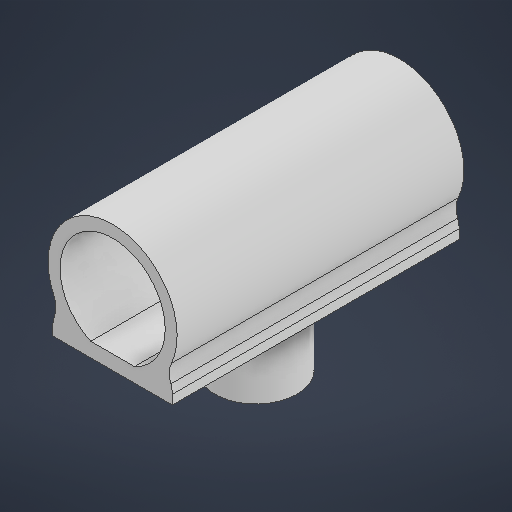
# Autodesk Inventor part: wire_loop
Saved by Autodesk Inventor 2027 (Build 310192060, 192F)
## iProperties
Created: 2026-07-23
Part Number: wire_loop
Material: Ogólny
Document SubType Name: Modeling
Designer: User
Density: 1 g/cm^3
Appearance: Domyślna
Author: User
Autodesk Inventor part; units mm, degrees
ref_plane "YZ Plane" through (0, 0, 0) normal (1, 0, 0) x (0, 1, 0)
ref_plane "XZ Plane" through (0, 0, 0) normal (0, 1, 0) x (-1, 0, 0)
ref_plane "XY Plane" through (0, 0, 0) normal (0, 0, 1) x (1, 0, 0)
sketch "Szkic1" plane through (0, 0, 0) normal (0, 1, 0) x (-1, 0, 0)
  circle A0 centre (0, 0) radius 1.72
  line L0 (-2.5, 6) -> (2.5, 6)
  line L1 (2.5, 6) -> (2.5, -6)
  line L2 (2.5, -6) -> (-2.5, -6)
  line L3 (-2.5, -6) -> (-2.5, 6)
  line L4 (-2.5, 6) -> (2.5, -6) construction
  line L5 (2.5, 6) -> (-2.5, -6) construction
  dimension "d0" = 3.44
  dimension "d1" = 5
  dimension "d2" = 12
  constraints: 12 end point, 2 midpoint, 2 parallel, 1 centre point, 1 coincident, 1 horizontal, 1 perpendicular
  measures "d0" diameter of A0
  measures "d1" distance of L1.end L2.end
  measures "d2" distance of L0.end L1.end
extrude "Wyciągnięcie proste1" add sketch "Szkic1" against normal blind 3 contours A0
extrude "Wyciągnięcie proste2" add sketch "Szkic1" along normal blind 0.6 contours A0 | L0 L1 L2 L3
sketch "Szkic2" plane through (-2.5, 0, 6) normal (0, 0, 1) x (1, 0, 0)
  line L0 (5, 0.6) -> (0, 0.6) projected
  line L1 (2.5, 0.6) -> (2.5, 2.6)
  line L2 (2.5, 0.6) -> (4.5, 0.6) construction
  circle A0 centre (2.5, 2.6) radius 2.2
  line L3 (0, 0.6) -> (5, 0.6)
  circle A1 centre (2.5, 2.6) radius 2.7
  point P0 (2.5, 0)
  point P1 (4.3138, 0.6)
  point P2 (0.6862, 0.6)
  point P3 (1.5835, 0.6)
  point P4 (3.4165, 0.6)
  dimension "d7" = 2
  dimension "d8" = 90
  dimension "d9" = 4.4
  dimension "d10" = 5.4
  constraints: 6 end point, 2 centre point, 2 coincident, 1 collinear, 1 horizontal, 1 midpoint, 1 perpendicular, 1 vertical
  measures "d7" distance of L1.start L1.end
  measures "d8" angle of L2 L1
  measures "d9" diameter of A0
  measures "d10" diameter of A1
extrude "Wyciągnięcie proste3" add sketch "Szkic2" against normal up to surface (12 mm away) contours L0 A0 A1 picked at (4.985, 2.9942)
fillet "Zaokrąglenie1" radius 1 4 edges at (1.8138, 0.6, 0) (-1.8138, 0.6, 0) (2.5, 0.6, 0) (-2.5, 0.6, 0)
